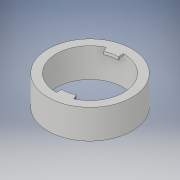
# Autodesk Inventor part: RSL light mount (guard 1)
Saved by Autodesk Inventor 2019 (Build 230136000, 136)
## iProperties
Created: 2019-02-13
Part Number: RSL light mount (guard 1)
Material: Generic
Document SubType Name: Modeling
Designer: josh
Density: 1 g/cm^3
Appearance: Default
Author: josh
Autodesk Inventor part; units mm, degrees
ref_plane "YZ Plane" through (0, 0, 0) normal (1, 0, 0) x (0, 1, 0)
ref_plane "XZ Plane" through (0, 0, 0) normal (0, 1, 0) x (-1, 0, 0)
sketch "Sketch1" plane through (0, 0, 0) normal (1, 0, 0) x (0, 1, 0)
  line L0 (-8.509, -17.279) -> (-10.287, -17.279)
  line L1 (-10.287, -17.279) -> (-10.287, -18.168)
  line L2 (-10.287, -18.168) -> (-9.398, -18.168)
  line L3 (-9.398, -18.168) -> (-9.398, -20.454)
  line L4 (-9.398, -20.454) -> (-8.509, -20.454)
  line L5 (-8.509, 20.454) -> (-8.509, 17.279)
  line L6 (-8.509, 17.279) -> (-10.287, 17.279)
  line L7 (-10.287, 17.279) -> (-10.287, 18.168)
  line L8 (-10.287, 18.168) -> (-9.398, 18.168)
  line L9 (-9.398, 18.168) -> (-9.398, 20.454)
  line L10 (-8.509, 20.454) -> (-8.509, 25.534)
  line L11 (-8.509, 25.534) -> (-26.289, 25.534)
  line L12 (-26.289, 25.534) -> (-26.289, 20.454)
  line L13 (-26.289, 20.454) -> (-9.398, 20.454)
  line L14 (-8.509, -20.454) -> (-8.509, -25.534)
  line L15 (-8.509, -25.534) -> (-26.289, -25.534)
  line L16 (-26.289, -25.534) -> (-26.289, -20.454)
  line L17 (-26.289, -20.454) -> (-9.398, -20.454)
  line L18 (-26.289, 20.454) -> (-23.749, 20.454)
  line L19 (-8.509, -17.279) -> (-8.509, -20.454)
  line L20 (-8.509, -17.279) -> (-8.509, 17.279)
  line L21 (-8.509, 0) -> (-26.289, 0)
  dimension "d8" = 1.778
  dimension "d10" = 0.889
  dimension "d13" = 0.889
  dimension "d15" = 17.78
  dimension "d16" = 5.08
  dimension "d17" = 17.78
  dimension "d18" = 2.54
  constraints: 44 end point, 8 perpendicular, 4 horizontal, 4 vertical, 1 collinear, 1 midpoint, 1 parallel, 1 point on line
  measures "d8" distance of L0.start L0.end
  measures "d10" distance of L0.end L1.end
  measures "d13" distance of L6.end L7.end
  measures "d15" distance of L10.end L11.end
  measures "d16" distance of L4.end L14.end
  measures "d17" distance of L14.end L15.end
  measures "d18" distance of L12.end L18.end
sketch "Sketch1 outline for Revolution1" plane through (0, 0, 0) normal (1, 0, 0) x (0, 1, 0)
  line L0 (-9.398, -18.168) -> (-9.398, -20.454)
  line L1 (-9.398, -20.454) -> (-26.289, -20.454)
  line L2 (-26.289, -20.454) -> (-26.289, -25.534)
  line L3 (-26.289, -25.534) -> (-8.509, -25.534)
  line L4 (-8.509, -25.534) -> (-8.509, -17.279)
  line L5 (-8.509, -17.279) -> (-10.287, -17.279)
  line L6 (-10.287, -17.279) -> (-10.287, -18.168)
  line L7 (-10.287, -18.168) -> (-9.398, -18.168)
  line L8 (-10.287, 17.279) -> (-8.509, 17.279)
  line L9 (-8.509, 17.279) -> (-8.509, 25.534)
  line L10 (-8.509, 25.534) -> (-26.289, 25.534)
  line L11 (-26.289, 25.534) -> (-26.289, 20.454)
  line L12 (-26.289, 20.454) -> (-9.398, 20.454)
  line L13 (-9.398, 20.454) -> (-9.398, 18.168)
  line L14 (-9.398, 18.168) -> (-10.287, 18.168)
  line L15 (-10.287, 18.168) -> (-10.287, 17.279)
revolve "Revolution1" add sketch "Sketch1 outline for Revolution1" angle 25 about axis through (0, -8.509, 0) along (0, 1, 0)
ref_plane "Work Plane1" through (0, -8.509, -25.534) normal (-1, 0, 0) x (0, -1, 0)
sketch "Sketch2" plane through (0, -8.509, -25.534) normal (-1, 0, 0) x (0, -1, 0)
  line L0 (0.889, 5.08) -> (17.78, 5.08)
  line L1 (17.78, 5.08) -> (17.78, 0)
  line L2 (0, 51.068) -> (17.78, 51.068)
  line L3 (17.78, 51.068) -> (0, 51.068)
  line L4 (-8.509, 25.534) -> (17.78, 25.534)
  line L5 (17.78, 51.068) -> (0, 51.068)
  line L6 (0, 51.068) -> (0, 45.988)
  line L7 (0, 45.988) -> (17.78, 45.988)
  line L8 (17.78, 45.988) -> (17.78, 51.068)
  line L9 (0.889, 5.08) -> (0, 5.08)
  line L10 (17.78, 5.08) -> (17.78, 0)
  line L11 (17.78, 2.392337) -> (17.78, 0)
  line L12 (17.78, 0) -> (0, 0)
  line L13 (0, 0) -> (0, 5.08)
  point P0 (0.889, 7.366)
  constraints: 22 end point, 3 perpendicular, 2 horizontal, 1 parallel
sketch "Sketch2 outline for Revolution2" plane through (0, -8.509, -25.534) normal (-1, 0, 0) x (0, -1, 0)
  line L0 (17.78, 5.08) -> (0, 5.08)
  line L1 (0, 5.08) -> (0, 0)
  line L2 (0, 0) -> (17.78, 0)
  line L3 (17.78, 0) -> (17.78, 5.08)
  line L4 (17.78, 45.988) -> (17.78, 51.068)
  line L5 (0, 45.988) -> (17.78, 45.988)
  line L6 (0, 51.068) -> (0, 45.988)
  line L7 (17.78, 51.068) -> (0, 51.068)
revolve "Revolution2" add sketch "Sketch2 outline for Revolution2" angle 155 about axis through (0, 0, 0) along (0, -1, 0)
body "Solid1"
